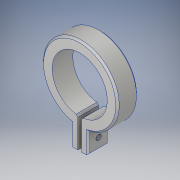
# Autodesk Inventor part: blocage_ressort_canon
Saved by Autodesk Inventor 2019 (Build 230136000, 136)
## iProperties
Created: 2019-03-26
Part Number: blocage_ressort_canon
Material: Aluminium 6061
Document SubType Name: Modeling
Designer: theor
Density: 2.7 g/cm^3
Appearance: Aluminium - Plat
Mass: 3.13666 g
Surface Area: 12.3917 cm^2
Volume: 1.16172 cm^3
Author: theor
Autodesk Inventor part; units mm, degrees
ref_plane "YZ Plane" through (0, 0, 0) normal (1, 0, 0) x (0, 1, 0)
ref_plane "XZ Plane" through (0, 0, 0) normal (0, 1, 0) x (-1, 0, 0)
ref_plane "XY Plane" through (0, 0, 0) normal (0, 0, 1) x (1, 0, 0)
sketch "Esquisse1" plane through (0, 0, 0) normal (0, 0, 1) x (1, 0, 0)
  arc A0 (0.5, -7.9844) -> (-0.5, -7.9844) centre (0, 0) ccw
  arc A1 (2.5, -10.7121) -> (-2.5, -10.7121) centre (0, 0) ccw
  line L0 (-0.5, -7.9844) -> (-0.5, -16.7121)
  line L1 (0.5, -7.9844) -> (0.5, -16.7121)
  line L2 (-0.5, -7.9844) -> (0.5, -7.9844) construction
  line L3 (-0.5, -16.7121) -> (-2.5, -16.7121)
  line L4 (-2.5, -16.7121) -> (-2.5, -10.7121)
  line L5 (0.5, -16.7121) -> (2.5, -16.7121)
  line L6 (2.5, -16.7121) -> (2.5, -10.7121)
  point P0 (0, -7.9844)
  dimension "d0" = 8
  dimension "d1" = 1
  dimension "d2" = 3
  dimension "d3" = 6
  dimension "d4" = 2
  constraints: 14 end point, 4 point on circle, 4 vertical, 3 horizontal, 2 centre point, 2 coincident, 2 collinear, 1 midpoint, 1 vertical alignment
  measures "d0" radius of A0
  measures "d1" distance of L0.start L1.start
  measures "d2" radial gap between concentric circles of A1 A0
  measures "d3" distance of L5.end L6.end
  measures "d4" distance of L1.end L5.end
extrude "Extrusion1" add sketch "Esquisse1" along normal blind 6
chamfer "Chanfrein1" distance 0.5 angle 45 10 edges at (0, 11, 6) (0, 11, 0) (-2.5, -16.7121, 3) (2.5, -16.7121, 3) (2.5, -13.7121, 6) (2.5, -13.7121, 0) (-2.5, -13.7121, 6) (-2.5, -13.7121, 0) (-0.5, -7.9844, 3) (0.5, -7.9844, 3)
sketch "Esquisse2" plane through (-2.5, -16.2121, 0.5) normal (-1, 0, 0) x (0, 0, 1)
  line L0 (-0.5, -0.5) -> (5.5, -0.5) projected
  line L1 (5.5, -0.5) -> (5.5, 5.9044) projected
  point P0 (-0.5, 16.2121)
  point P1 (2.5, 2.7022)
  point P2 (2.5, -0.5)
  point P3 (5.5, 2.7022)
  constraints: 2 midpoint, 1 horizontal alignment, 1 vertical alignment
hole "Perçage1" at (-2.5, -13.51, 3) direction (1, 0, 0) diameter 2.4 depth 2 clearance for "Vis d'assemblage à six pans creux ISO 4762" size "M2" standard "ISO"
sketch "Esquisse3" plane through (2.5, -16.2121, 0.5) normal (1, 0, 0) x (0, 0, -1)
  line L0 (0.5, -0.5) -> (0.5, 5.9044) projected
  line L1 (-5.5, -0.5) -> (0.5, -0.5) projected
  point P0 (0.5, 16.2121)
  point P1 (-2.5, 2.7022)
  point P2 (0.5, 2.7022)
  point P3 (-2.5, -0.5)
  constraints: 2 midpoint, 1 horizontal alignment, 1 vertical alignment
hole "Perçage2" at (2.5, -13.51, 3) direction (-1, 0, 0) diameter 1.567 depth 2 thread size "M2x0.4" class "6H" standard "ISO Metric profile"
